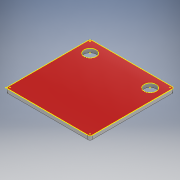
# Autodesk Inventor part: RGBsensor
Saved by Autodesk Inventor 2017 (Build 210142000, 142)
## iProperties
Created: 2017-12-13
Part Number: RGBsensor
Material: Generic
Document SubType Name: Modeling
Designer: Carolina Lema
Density: 1 g/cm^3
Appearance: Default
Author: Carolina Lema
Autodesk Inventor part; units mm, degrees
ref_plane "YZ Plane" through (0, 0, 0) normal (1, 0, 0) x (0, 1, 0)
ref_plane "XZ Plane" through (0, 0, 0) normal (0, 1, 0) x (-1, 0, 0)
ref_plane "XY Plane" through (0, 0, 0) normal (0, 0, 1) x (1, 0, 0)
sketch "Sketch1" plane through (0, 0, 0) normal (0, 0, 1) x (1, 0, 0)
  line L0 (0.5, 0) -> (20.5, 0)
  line L1 (21, 0.5) -> (21, 20.5)
  line L2 (20.5, 21) -> (0.5, 21)
  line L3 (0, 20.5) -> (0, 0.5)
  line L4 (0, 20.5) -> (0, 20)
  line L5 (1, 21) -> (0.5, 21)
  line L6 (0, 1) -> (0, 0.5)
  line L7 (0.5, 0) -> (1, 0)
  line L8 (21, 20) -> (21, 20.5)
  line L9 (20.5, 21) -> (20, 21)
  line L10 (20, 0) -> (20.5, 0)
  line L11 (21, 0.5) -> (21, 1)
  arc A0 (0.5, 21) -> (0, 20.5) centre (0.5, 20.5) ccw
  arc A1 (21, 20.5) -> (20.5, 21) centre (20.5, 20.5) ccw
  arc A2 (20.5, 0) -> (21, 0.5) centre (20.5, 0.5) ccw
  arc A3 (0, 0.5) -> (0.5, 0) centre (0.5, 0.5) ccw
  line L12 (0, 21) -> (0, 19.5)
  line L13 (0, 19.5) -> (3, 19.5)
  line L14 (21, 21) -> (21, 19.5)
  line L15 (21, 19.5) -> (18, 19.5)
  line L16 (3, 19.5) -> (3, 18)
  line L17 (18, 19.5) -> (18, 18)
  circle A4 centre (3, 18) radius 1.5
  circle A5 centre (18, 18) radius 1.5
  point P0 (0, 0)
  dimension "d4" = 1.5
  dimension "d5" = 3
  dimension "d6" = 1.5
  dimension "d7" = 3
  dimension "d8" = 1.5
  dimension "d9" = 1.5
  constraints: 36 end point, 8 point on circle, 5 point on line, 4 centre point, 4 perpendicular, 4 tangent, 2 coincident, 2 parallel, 2 vertical, 2 vertical alignment, 1 collinear, 1 horizontal, 4 other
  measures "d4" distance of L12.start L12.end
  measures "d5" distance of L12.end L13.end
  measures "d6" distance of L14.start L14.end
  measures "d7" distance of L14.end L15.end
  measures "d8" distance of L13.end L16.end
  measures "d9" distance of L15.end L17.end
extrude "Extrusion1" add sketch "Sketch1" along normal blind 1
sketch "Sketch2" plane through (0, 0, 1) normal (0, 0, 1) x (1, 0, 0)
  line L0 (20.5, 21) -> (0.5, 21) projected
  circle A0 centre (18, 18) radius 1.5 projected
  circle A1 centre (3, 18) radius 1.5 projected
  line L1 (20.5, 21) -> (0.5, 21) projected
  arc A2 (0.5, 21) -> (0, 20.5) centre (0.5, 20.5) ccw projected
  line L2 (0, 20.5) -> (0, 0.5) projected
  arc A3 (0, 0.5) -> (0.5, 0) centre (0.5, 0.5) ccw projected
  line L3 (0.5, 0) -> (20.5, 0) projected
  arc A4 (20.5, 0) -> (21, 0.5) centre (20.5, 0.5) ccw projected
  line L4 (21, 0.5) -> (21, 20.5) projected
  arc A5 (21, 20.5) -> (20.5, 21) centre (20.5, 20.5) ccw projected
  point P0 (0, 0)
body "Solid1"
